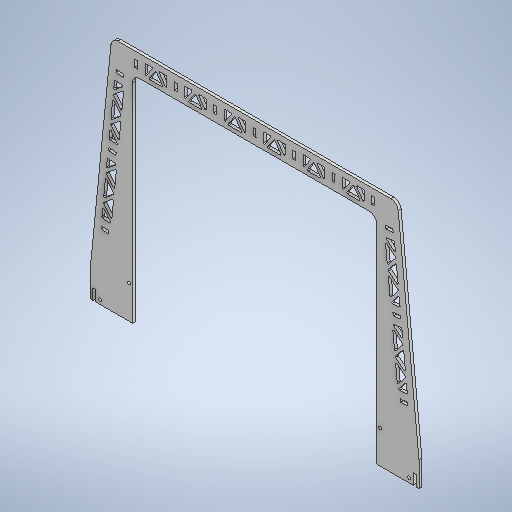
# Autodesk Inventor part: GateBrigeSide
Saved by Autodesk Inventor 2025.1 (Build 291241000, 241)
## iProperties
Created: 2025-03-30
Part Number: GateBrigeSide
Material: Všeobecné
Document SubType Name: Modeling
Designer: 42060
Density: 1 g/cm^3
Appearance: Výchozí
Author: 42060
Autodesk Inventor part; units mm, degrees
ref_plane "YZ Plane" through (0, 0, 0) normal (1, 0, 0) x (0, 1, 0)
ref_plane "XZ Plane" through (0, 0, 0) normal (0, 1, 0) x (-1, 0, 0)
ref_plane "XY Plane" through (0, 0, 0) normal (0, 0, 1) x (1, 0, 0)
sketch "Náčrt1" plane through (0, 0, 0) normal (0, 0, 1) x (1, 0, 0)
  line L0 (0, 0) -> (-160, 0)
  line L1 (-170, -10) -> (-170, -300)
  line L2 (-229, -300) -> (-229, -265.3)
  line L3 (-190.0509, 30) -> (0, 30)
  line L4 (0, 30) -> (0, 0)
  line L5 (-203.7, -249) -> (-170, -249)
  line L6 (-170, -249) -> (-170, -299)
  line L7 (-170, -299) -> (-220, -299)
  line L8 (-220, -299) -> (-220, -265.3)
  line L9 (-220, -265.3) -> (-203.7, -249)
  line L10 (-220, -299) -> (-170, -249) construction
  circle A0 centre (-215, -294) radius 2.1
  circle A1 centre (-175, -254) radius 2.1
  arc A2 (-160, 0) -> (-170, -10) centre (-160, -10) ccw
  line L11 (-200, 21.0077) -> (-229, -265.3)
  arc A3 (-190.0509, 30) -> (-200, 21.0077) centre (-190.0509, 20) ccw
  line L12 (-225, -300) -> (-225, -285)
  line L13 (-225, -285) -> (-221, -285)
  line L14 (-221, -285) -> (-221, -300)
  line L15 (-170, -300) -> (-221, -300)
  line L16 (-225, -300) -> (-229, -300)
  line L17 (-2, 10) -> (2, 10)
  line L18 (2, 10) -> (2, 20)
  line L19 (2, 20) -> (-2, 20)
  line L20 (-2, 20) -> (-2, 10)
  line L21 (-57, 20) -> (-57, 10)
  line L22 (-53, 20) -> (-57, 20)
  line L23 (-53, 10) -> (-53, 20)
  line L24 (-57, 10) -> (-53, 10)
  line L25 (-112, 20) -> (-112, 10)
  line L26 (-108, 20) -> (-112, 20)
  line L27 (-108, 10) -> (-108, 20)
  line L28 (-112, 10) -> (-108, 10)
  line L29 (-167, 20) -> (-167, 10)
  line L30 (-163, 20) -> (-167, 20)
  line L31 (-163, 10) -> (-163, 20)
  line L32 (-167, 10) -> (-163, 10)
  line L33 (-192.5844, -5.0126) -> (-182.6353, -6.0204)
  line L34 (-182.6353, -6.0204) -> (-183.0384, -10)
  line L35 (-183.0384, -10) -> (-192.9875, -8.9923)
  line L36 (-192.9875, -8.9923) -> (-192.5844, -5.0126)
  line L37 (-193.1158, -109.4909) -> (-203.0649, -108.4832)
  line L38 (-192.7127, -105.5113) -> (-193.1158, -109.4909)
  line L39 (-203.0649, -108.4832) -> (-202.6618, -104.5036)
  line L40 (-202.6618, -104.5036) -> (-192.7127, -105.5113)
  line L41 (-203.1932, -208.9819) -> (-213.1423, -207.9741)
  line L42 (-202.7901, -205.0022) -> (-203.1932, -208.9819)
  line L43 (-213.1423, -207.9741) -> (-212.7392, -203.9945)
  line L44 (-212.7392, -203.9945) -> (-202.7901, -205.0022)
  line L45 (0, 0) -> (160, 0)
  line L46 (170, -10) -> (170, -300)
  line L47 (229, -300) -> (229, -265.3)
  line L48 (190.0509, 30) -> (0, 30)
  line L49 (203.7, -249) -> (170, -249)
  line L50 (170, -249) -> (170, -299)
  line L51 (170, -299) -> (220, -299)
  line L52 (220, -299) -> (220, -265.3)
  line L53 (220, -265.3) -> (203.7, -249)
  line L54 (220, -299) -> (170, -249) construction
  circle A4 centre (215, -294) radius 2.1
  circle A5 centre (175, -254) radius 2.1
  arc A6 (170, -10) -> (160, 0) centre (160, -10) ccw
  line L55 (200, 21.0077) -> (229, -265.3)
  arc A7 (200, 21.0077) -> (190.0509, 30) centre (190.0509, 20) ccw
  line L56 (225, -300) -> (225, -285)
  line L57 (225, -285) -> (221, -285)
  line L58 (221, -285) -> (221, -300)
  line L59 (170, -300) -> (221, -300)
  line L60 (225, -300) -> (229, -300)
  line L61 (2, 10) -> (-2, 10)
  line L62 (-2, 10) -> (-2, 20)
  line L63 (-2, 20) -> (2, 20)
  line L64 (2, 20) -> (2, 10)
  line L65 (57, 20) -> (57, 10)
  line L66 (53, 20) -> (57, 20)
  line L67 (53, 10) -> (53, 20)
  line L68 (57, 10) -> (53, 10)
  line L69 (112, 20) -> (112, 10)
  line L70 (108, 20) -> (112, 20)
  line L71 (108, 10) -> (108, 20)
  line L72 (112, 10) -> (108, 10)
  line L73 (167, 20) -> (167, 10)
  line L74 (163, 20) -> (167, 20)
  line L75 (163, 10) -> (163, 20)
  line L76 (167, 10) -> (163, 10)
  line L77 (192.5844, -5.0126) -> (182.6353, -6.0204)
  line L78 (182.6353, -6.0204) -> (183.0384, -10)
  line L79 (183.0384, -10) -> (192.9875, -8.9923)
  line L80 (192.9875, -8.9923) -> (192.5844, -5.0126)
  line L81 (193.1158, -109.4909) -> (203.0649, -108.4832)
  line L82 (192.7127, -105.5113) -> (193.1158, -109.4909)
  line L83 (203.0649, -108.4832) -> (202.6618, -104.5036)
  line L84 (202.6618, -104.5036) -> (192.7127, -105.5113)
  line L85 (203.1932, -208.9819) -> (213.1423, -207.9741)
  line L86 (202.7901, -205.0022) -> (203.1932, -208.9819)
  line L87 (213.1423, -207.9741) -> (212.7392, -203.9945)
  line L88 (212.7392, -203.9945) -> (202.7901, -205.0022)
  line L89 (-36.6095, 7.1947) -> (-28.3278, 19.4124)
  line L90 (-26.6722, 19.4124) -> (-18.3905, 7.1947)
  line L91 (-19.2183, 5.6336) -> (-35.7817, 5.6336)
  line L92 (-22.6095, 20.5478) -> (-14.3278, 8.33)
  line L93 (-12.5, 8.8911) -> (-12.5, 21.1089)
  line L94 (-13.5, 22.1089) -> (-21.7817, 22.1089)
  line L95 (-32.3905, 20.5478) -> (-40.6722, 8.33)
  line L96 (-42.5, 8.8911) -> (-42.5, 21.1089)
  line L97 (-41.5, 22.1089) -> (-33.2183, 22.1089)
  line L98 (-53, 15) -> (-2, 15) construction
  arc A8 (-41.5, 22.1089) -> (-42.5, 21.1089) centre (-41.5, 21.1089) ccw
  arc A9 (-32.3905, 20.5478) -> (-33.2183, 22.1089) centre (-33.2183, 21.1089) ccw
  arc A10 (-42.5, 8.8911) -> (-40.6722, 8.33) centre (-41.5, 8.8911) ccw
  arc A11 (-36.6095, 7.1947) -> (-35.7817, 5.6336) centre (-35.7817, 6.6336) ccw
  arc A12 (-19.2183, 5.6336) -> (-18.3905, 7.1947) centre (-19.2183, 6.6336) ccw
  arc A13 (-26.6722, 19.4124) -> (-28.3278, 19.4124) centre (-27.5, 18.8514) ccw
  arc A14 (-21.7817, 22.1089) -> (-22.6095, 20.5478) centre (-21.7817, 21.1089) ccw
  arc A15 (-12.5, 21.1089) -> (-13.5, 22.1089) centre (-13.5, 21.1089) ccw
  arc A16 (-14.3278, 8.33) -> (-12.5, 8.8911) centre (-13.5, 8.8911) ccw
  arc A17 (-81.6722, 19.4124) -> (-83.3278, 19.4124) centre (-82.5, 18.8514) ccw
  line L99 (-91.6095, 7.1947) -> (-83.3278, 19.4124)
  line L100 (-68.5, 22.1089) -> (-76.7817, 22.1089)
  arc A18 (-67.5, 21.1089) -> (-68.5, 22.1089) centre (-68.5, 21.1089) ccw
  line L101 (-81.6722, 19.4124) -> (-73.3905, 7.1947)
  arc A19 (-74.2183, 5.6336) -> (-73.3905, 7.1947) centre (-74.2183, 6.6336) ccw
  line L102 (-77.6095, 20.5478) -> (-69.3278, 8.33)
  line L103 (-74.2183, 5.6336) -> (-90.7817, 5.6336)
  arc A20 (-69.3278, 8.33) -> (-67.5, 8.8911) centre (-68.5, 8.8911) ccw
  line L104 (-108, 15) -> (-57, 15) construction
  arc A21 (-96.5, 22.1089) -> (-97.5, 21.1089) centre (-96.5, 21.1089) ccw
  arc A22 (-97.5, 8.8911) -> (-95.6722, 8.33) centre (-96.5, 8.8911) ccw
  arc A23 (-91.6095, 7.1947) -> (-90.7817, 5.6336) centre (-90.7817, 6.6336) ccw
  arc A24 (-87.3905, 20.5478) -> (-88.2183, 22.1089) centre (-88.2183, 21.1089) ccw
  line L105 (-67.5, 8.8911) -> (-67.5, 21.1089)
  arc A25 (-76.7817, 22.1089) -> (-77.6095, 20.5478) centre (-76.7817, 21.1089) ccw
  line L106 (-96.5, 22.1089) -> (-88.2183, 22.1089)
  line L107 (-87.3905, 20.5478) -> (-95.6722, 8.33)
  line L108 (-97.5, 8.8911) -> (-97.5, 21.1089)
  arc A26 (-136.6722, 19.4124) -> (-138.3278, 19.4124) centre (-137.5, 18.8514) ccw
  line L109 (-146.6095, 7.1947) -> (-138.3278, 19.4124)
  line L110 (-123.5, 22.1089) -> (-131.7817, 22.1089)
  arc A27 (-122.5, 21.1089) -> (-123.5, 22.1089) centre (-123.5, 21.1089) ccw
  line L111 (-136.6722, 19.4124) -> (-128.3905, 7.1947)
  arc A28 (-129.2183, 5.6336) -> (-128.3905, 7.1947) centre (-129.2183, 6.6336) ccw
  line L112 (-132.6095, 20.5478) -> (-124.3278, 8.33)
  line L113 (-129.2183, 5.6336) -> (-145.7817, 5.6336)
  arc A29 (-124.3278, 8.33) -> (-122.5, 8.8911) centre (-123.5, 8.8911) ccw
  line L114 (-163, 15) -> (-112, 15) construction
  arc A30 (-151.5, 22.1089) -> (-152.5, 21.1089) centre (-151.5, 21.1089) ccw
  arc A31 (-152.5, 8.8911) -> (-150.6722, 8.33) centre (-151.5, 8.8911) ccw
  arc A32 (-146.6095, 7.1947) -> (-145.7817, 5.6336) centre (-145.7817, 6.6336) ccw
  arc A33 (-142.3905, 20.5478) -> (-143.2183, 22.1089) centre (-143.2183, 21.1089) ccw
  line L115 (-122.5, 8.8911) -> (-122.5, 21.1089)
  arc A34 (-131.7817, 22.1089) -> (-132.6095, 20.5478) centre (-131.7817, 21.1089) ccw
  line L116 (-151.5, 22.1089) -> (-143.2183, 22.1089)
  line L117 (-142.3905, 20.5478) -> (-150.6722, 8.33)
  line L118 (-152.5, 8.8911) -> (-152.5, 21.1089)
  line L119 (-193.9599, -18.9449) -> (-184.0815, -19.9455)
  line L120 (-183.55, -21.7152) -> (-194.429, -30.593)
  line L121 (-196.0562, -29.7175) -> (-195.0556, -19.8391)
  line L122 (-182.493, -28.2188) -> (-184.6957, -49.9654)
  line L123 (-186.4653, -50.4969) -> (-196.2373, -38.5222)
  line L124 (-196.0948, -37.1152) -> (-184.1201, -27.3432)
  line L125 (-195.9132, -45.2459) -> (-186.1413, -57.2206)
  line L126 (-186.2838, -58.6276) -> (-198.2584, -68.3996)
  line L127 (-199.8856, -67.524) -> (-197.6829, -45.7774)
  line L128 (-187.9495, -65.1498) -> (-199.9242, -74.9217)
  line L129 (-200.0667, -76.3288) -> (-190.2947, -88.3034)
  line L130 (-188.5251, -87.7719) -> (-186.3224, -66.0253)
  line L131 (-199.7426, -83.0525) -> (-190.8648, -93.9315)
  line L132 (-191.7403, -95.5586) -> (-201.6187, -94.558)
  line L133 (-202.5129, -93.4624) -> (-201.5123, -83.584)
  line L134 (-189.0207, -19.4452) -> (-188.013, -9.4961)
  arc A35 (-193.9599, -18.9449) -> (-195.0556, -19.8391) centre (-194.0607, -19.9398) ccw
  arc A36 (-183.55, -21.7152) -> (-184.0815, -19.9455) centre (-184.1823, -20.9404) ccw
  arc A37 (-196.0562, -29.7175) -> (-194.429, -30.593) centre (-195.0613, -29.8182) ccw
  arc A38 (-196.0948, -37.1152) -> (-196.2373, -38.5222) centre (-195.4625, -37.89) ccw
  arc A39 (-186.4653, -50.4969) -> (-184.6957, -49.9654) centre (-185.6906, -49.8646) ccw
  arc A40 (-182.493, -28.2188) -> (-184.1201, -27.3432) centre (-183.4879, -28.118) ccw
  arc A41 (-195.9132, -45.2459) -> (-197.6829, -45.7774) centre (-196.688, -45.8782) ccw
  arc A42 (-186.2838, -58.6276) -> (-186.1413, -57.2206) centre (-186.916, -57.8528) ccw
  arc A43 (-199.8856, -67.524) -> (-198.2584, -68.3996) centre (-198.8907, -67.6248) ccw
  arc A44 (-199.9242, -74.9217) -> (-200.0667, -76.3288) centre (-199.2919, -75.6965) ccw
  arc A45 (-190.2947, -88.3034) -> (-188.5251, -87.7719) centre (-189.52, -87.6712) ccw
  arc A46 (-186.3224, -66.0253) -> (-187.9495, -65.1498) centre (-187.3173, -65.9246) ccw
  arc A47 (-199.7426, -83.0525) -> (-201.5123, -83.584) centre (-200.5174, -83.6847) ccw
  arc A48 (-202.5129, -93.4624) -> (-201.6187, -94.558) centre (-201.518, -93.5631) ccw
  arc A49 (-191.7403, -95.5586) -> (-190.8648, -93.9315) centre (-191.6396, -94.5637) ccw
  arc A50 (-212.5903, -192.9533) -> (-211.6961, -194.049) centre (-211.5954, -193.0541) ccw
  line L135 (-201.8177, -195.0496) -> (-211.6961, -194.049)
  arc A51 (-201.8177, -195.0496) -> (-200.9422, -193.4224) centre (-201.717, -194.0546) ccw
  arc A52 (-200.3721, -187.7943) -> (-198.6025, -187.2629) centre (-199.5974, -187.1621) ccw
  line L136 (-209.82, -182.5434) -> (-200.9422, -193.4224)
  line L137 (-212.5903, -192.9533) -> (-211.5897, -183.0749)
  arc A53 (-209.82, -182.5434) -> (-211.5897, -183.0749) centre (-210.5948, -183.1757) ccw
  line L138 (-198.0269, -164.6407) -> (-210.0016, -174.4127)
  line L139 (-210.1441, -175.8197) -> (-200.3721, -187.7943)
  line L140 (-198.6025, -187.2629) -> (-196.3998, -165.5163)
  arc A54 (-210.0016, -174.4127) -> (-210.1441, -175.8197) centre (-209.3693, -175.1874) ccw
  arc A55 (-209.963, -167.0149) -> (-208.3358, -167.8905) centre (-208.9681, -167.1157) ccw
  arc A56 (-196.3998, -165.5163) -> (-198.0269, -164.6407) centre (-197.3947, -165.4155) ccw
  line L141 (-205.9906, -144.7369) -> (-196.2187, -156.7115)
  arc A57 (-196.3612, -158.1185) -> (-196.2187, -156.7115) centre (-196.9934, -157.3438) ccw
  line L142 (-209.963, -167.0149) -> (-207.7603, -145.2684)
  line L143 (-196.3612, -158.1185) -> (-208.3358, -167.8905)
  arc A58 (-196.5427, -149.9878) -> (-194.7731, -149.4563) centre (-195.768, -149.3555) ccw
  arc A59 (-205.9906, -144.7369) -> (-207.7603, -145.2684) centre (-206.7654, -145.3691) ccw
  line L144 (-196.5427, -149.9878) -> (-206.3147, -138.0131)
  arc A60 (-206.1722, -136.6061) -> (-206.3147, -138.0131) centre (-205.5399, -137.3809) ccw
  arc A61 (-206.1336, -129.2084) -> (-204.5064, -130.0839) centre (-205.1387, -129.3092) ccw
  line L145 (-192.5703, -127.7097) -> (-194.7731, -149.4563)
  line L146 (-206.1722, -136.6061) -> (-194.1975, -126.8342)
  arc A62 (-192.5703, -127.7097) -> (-194.1975, -126.8342) centre (-193.5653, -127.6089) ccw
  arc A63 (-193.6274, -121.2061) -> (-194.1589, -119.4364) centre (-194.2597, -120.4314) ccw
  line L147 (-199.0981, -118.9362) -> (-198.0904, -108.9871)
  line L148 (-204.0373, -118.4359) -> (-194.1589, -119.4364)
  arc A64 (-204.0373, -118.4359) -> (-205.133, -119.33) centre (-204.1381, -119.4308) ccw
  line L149 (-193.6274, -121.2061) -> (-204.5064, -130.0839)
  line L150 (-206.1336, -129.2084) -> (-205.133, -119.33)
  line L151 (36.6095, 7.1947) -> (28.3278, 19.4124)
  line L152 (26.6722, 19.4124) -> (18.3905, 7.1947)
  line L153 (19.2183, 5.6336) -> (35.7817, 5.6336)
  line L154 (22.6095, 20.5478) -> (14.3278, 8.33)
  line L155 (12.5, 8.8911) -> (12.5, 21.1089)
  line L156 (13.5, 22.1089) -> (21.7817, 22.1089)
  line L157 (32.3905, 20.5478) -> (40.6722, 8.33)
  line L158 (42.5, 8.8911) -> (42.5, 21.1089)
  line L159 (41.5, 22.1089) -> (33.2183, 22.1089)
  line L160 (53, 15) -> (2, 15) construction
  arc A65 (42.5, 21.1089) -> (41.5, 22.1089) centre (41.5, 21.1089) ccw
  arc A66 (33.2183, 22.1089) -> (32.3905, 20.5478) centre (33.2183, 21.1089) ccw
  arc A67 (40.6722, 8.33) -> (42.5, 8.8911) centre (41.5, 8.8911) ccw
  arc A68 (35.7817, 5.6336) -> (36.6095, 7.1947) centre (35.7817, 6.6336) ccw
  arc A69 (18.3905, 7.1947) -> (19.2183, 5.6336) centre (19.2183, 6.6336) ccw
  arc A70 (28.3278, 19.4124) -> (26.6722, 19.4124) centre (27.5, 18.8514) ccw
  arc A71 (22.6095, 20.5478) -> (21.7817, 22.1089) centre (21.7817, 21.1089) ccw
  arc A72 (13.5, 22.1089) -> (12.5, 21.1089) centre (13.5, 21.1089) ccw
  arc A73 (12.5, 8.8911) -> (14.3278, 8.33) centre (13.5, 8.8911) ccw
  line L161 (67.5, 8.8911) -> (67.5, 21.1089)
  line L162 (96.5, 22.1089) -> (88.2183, 22.1089)
  arc A74 (97.5, 21.1089) -> (96.5, 22.1089) centre (96.5, 21.1089) ccw
  line L163 (97.5, 8.8911) -> (97.5, 21.1089)
  arc A75 (95.6722, 8.33) -> (97.5, 8.8911) centre (96.5, 8.8911) ccw
  arc A76 (67.5, 8.8911) -> (69.3278, 8.33) centre (68.5, 8.8911) ccw
  arc A77 (68.5, 22.1089) -> (67.5, 21.1089) centre (68.5, 21.1089) ccw
  arc A78 (88.2183, 22.1089) -> (87.3905, 20.5478) centre (88.2183, 21.1089) ccw
  arc A79 (83.3278, 19.4124) -> (81.6722, 19.4124) centre (82.5, 18.8514) ccw
  line L164 (87.3905, 20.5478) -> (95.6722, 8.33)
  line L165 (91.6095, 7.1947) -> (83.3278, 19.4124)
  arc A80 (77.6095, 20.5478) -> (76.7817, 22.1089) centre (76.7817, 21.1089) ccw
  arc A81 (90.7817, 5.6336) -> (91.6095, 7.1947) centre (90.7817, 6.6336) ccw
  line L166 (108, 15) -> (57, 15) construction
  line L167 (68.5, 22.1089) -> (76.7817, 22.1089)
  line L168 (77.6095, 20.5478) -> (69.3278, 8.33)
  line L169 (81.6722, 19.4124) -> (73.3905, 7.1947)
  arc A82 (73.3905, 7.1947) -> (74.2183, 5.6336) centre (74.2183, 6.6336) ccw
  line L170 (74.2183, 5.6336) -> (90.7817, 5.6336)
  line L171 (122.5, 8.8911) -> (122.5, 21.1089)
  line L172 (151.5, 22.1089) -> (143.2183, 22.1089)
  arc A83 (152.5, 21.1089) -> (151.5, 22.1089) centre (151.5, 21.1089) ccw
  line L173 (152.5, 8.8911) -> (152.5, 21.1089)
  arc A84 (150.6722, 8.33) -> (152.5, 8.8911) centre (151.5, 8.8911) ccw
  arc A85 (122.5, 8.8911) -> (124.3278, 8.33) centre (123.5, 8.8911) ccw
  arc A86 (123.5, 22.1089) -> (122.5, 21.1089) centre (123.5, 21.1089) ccw
  arc A87 (143.2183, 22.1089) -> (142.3905, 20.5478) centre (143.2183, 21.1089) ccw
  arc A88 (138.3278, 19.4124) -> (136.6722, 19.4124) centre (137.5, 18.8514) ccw
  line L174 (142.3905, 20.5478) -> (150.6722, 8.33)
  line L175 (146.6095, 7.1947) -> (138.3278, 19.4124)
  arc A89 (132.6095, 20.5478) -> (131.7817, 22.1089) centre (131.7817, 21.1089) ccw
  arc A90 (145.7817, 5.6336) -> (146.6095, 7.1947) centre (145.7817, 6.6336) ccw
  line L176 (163, 15) -> (112, 15) construction
  line L177 (123.5, 22.1089) -> (131.7817, 22.1089)
  line L178 (132.6095, 20.5478) -> (124.3278, 8.33)
  line L179 (136.6722, 19.4124) -> (128.3905, 7.1947)
  arc A91 (128.3905, 7.1947) -> (129.2183, 5.6336) centre (129.2183, 6.6336) ccw
  line L180 (129.2183, 5.6336) -> (145.7817, 5.6336)
  line L181 (193.9599, -18.9449) -> (184.0815, -19.9455)
  line L182 (183.55, -21.7152) -> (194.429, -30.593)
  line L183 (196.0562, -29.7175) -> (195.0556, -19.8391)
  line L184 (182.493, -28.2188) -> (184.6957, -49.9654)
  line L185 (186.4653, -50.4969) -> (196.2373, -38.5222)
  line L186 (196.0948, -37.1152) -> (184.1201, -27.3432)
  line L187 (195.9132, -45.2459) -> (186.1413, -57.2206)
  line L188 (186.2838, -58.6276) -> (198.2584, -68.3996)
  line L189 (199.8856, -67.524) -> (197.6829, -45.7774)
  line L190 (187.9495, -65.1498) -> (199.9242, -74.9217)
  line L191 (200.0667, -76.3288) -> (190.2947, -88.3034)
  line L192 (188.5251, -87.7719) -> (186.3224, -66.0253)
  line L193 (199.7426, -83.0525) -> (190.8648, -93.9315)
  line L194 (191.7403, -95.5586) -> (201.6187, -94.558)
  line L195 (202.5129, -93.4624) -> (201.5123, -83.584)
  line L196 (189.0207, -19.4452) -> (188.013, -9.4961)
  arc A92 (195.0556, -19.8391) -> (193.9599, -18.9449) centre (194.0607, -19.9398) ccw
  arc A93 (184.0815, -19.9455) -> (183.55, -21.7152) centre (184.1823, -20.9404) ccw
  arc A94 (194.429, -30.593) -> (196.0562, -29.7175) centre (195.0613, -29.8182) ccw
  arc A95 (196.2373, -38.5222) -> (196.0948, -37.1152) centre (195.4625, -37.89) ccw
  arc A96 (184.6957, -49.9654) -> (186.4653, -50.4969) centre (185.6906, -49.8646) ccw
  arc A97 (184.1201, -27.3432) -> (182.493, -28.2188) centre (183.4879, -28.118) ccw
  arc A98 (197.6829, -45.7774) -> (195.9132, -45.2459) centre (196.688, -45.8782) ccw
  arc A99 (186.1413, -57.2206) -> (186.2838, -58.6276) centre (186.916, -57.8528) ccw
  arc A100 (198.2584, -68.3996) -> (199.8856, -67.524) centre (198.8907, -67.6248) ccw
  arc A101 (200.0667, -76.3288) -> (199.9242, -74.9217) centre (199.2919, -75.6965) ccw
  arc A102 (188.5251, -87.7719) -> (190.2947, -88.3034) centre (189.52, -87.6712) ccw
  arc A103 (187.9495, -65.1498) -> (186.3224, -66.0253) centre (187.3173, -65.9246) ccw
  arc A104 (201.5123, -83.584) -> (199.7426, -83.0525) centre (200.5174, -83.6847) ccw
  arc A105 (201.6187, -94.558) -> (202.5129, -93.4624) centre (201.518, -93.5631) ccw
  arc A106 (190.8648, -93.9315) -> (191.7403, -95.5586) centre (191.6396, -94.5637) ccw
  arc A107 (194.1589, -119.4364) -> (193.6274, -121.2061) centre (194.2597, -120.4314) ccw
  arc A108 (194.1975, -126.8342) -> (192.5703, -127.7097) centre (193.5653, -127.6089) ccw
  line L197 (204.0373, -118.4359) -> (194.1589, -119.4364)
  line L198 (193.6274, -121.2061) -> (204.5064, -130.0839)
  line L199 (206.1336, -129.2084) -> (205.133, -119.33)
  line L200 (206.1722, -136.6061) -> (194.1975, -126.8342)
  arc A109 (205.133, -119.33) -> (204.0373, -118.4359) centre (204.1381, -119.4308) ccw
  arc A110 (204.5064, -130.0839) -> (206.1336, -129.2084) centre (205.1387, -129.3092) ccw
  line L201 (192.5703, -127.7097) -> (194.7731, -149.4563)
  arc A111 (207.7603, -145.2684) -> (205.9906, -144.7369) centre (206.7654, -145.3691) ccw
  line L202 (196.5427, -149.9878) -> (206.3147, -138.0131)
  arc A112 (206.3147, -138.0131) -> (206.1722, -136.6061) centre (205.5399, -137.3809) ccw
  arc A113 (194.7731, -149.4563) -> (196.5427, -149.9878) centre (195.768, -149.3555) ccw
  line L203 (205.9906, -144.7369) -> (196.2187, -156.7115)
  arc A114 (196.2187, -156.7115) -> (196.3612, -158.1185) centre (196.9934, -157.3438) ccw
  arc A115 (198.0269, -164.6407) -> (196.3998, -165.5163) centre (197.3947, -165.4155) ccw
  line L204 (196.3612, -158.1185) -> (208.3358, -167.8905)
  arc A116 (208.3358, -167.8905) -> (209.963, -167.0149) centre (208.9681, -167.1157) ccw
  line L205 (209.963, -167.0149) -> (207.7603, -145.2684)
  arc A117 (200.9422, -193.4224) -> (201.8177, -195.0496) centre (201.717, -194.0546) ccw
  arc A118 (211.6961, -194.049) -> (212.5903, -192.9533) centre (211.5954, -193.0541) ccw
  arc A119 (198.6025, -187.2629) -> (200.3721, -187.7943) centre (199.5974, -187.1621) ccw
  line L206 (212.5903, -192.9533) -> (211.5897, -183.0749)
  line L207 (209.82, -182.5434) -> (200.9422, -193.4224)
  arc A120 (211.5897, -183.0749) -> (209.82, -182.5434) centre (210.5948, -183.1757) ccw
  line L208 (210.1441, -175.8197) -> (200.3721, -187.7943)
  arc A121 (210.1441, -175.8197) -> (210.0016, -174.4127) centre (209.3693, -175.1874) ccw
  line L209 (198.6025, -187.2629) -> (196.3998, -165.5163)
  line L210 (198.0269, -164.6407) -> (210.0016, -174.4127)
  line L211 (201.8177, -195.0496) -> (211.6961, -194.049)
  point P0 (2, 15)
  point P1 (0, 15)
  point P2 (0, 10)
  point P3 (-55, 10)
  point P4 (-110, 10)
  point P5 (-165, 10)
  point P6 (55, 10)
  point P7 (108, 15)
  point P8 (110, 10)
  point P9 (163, 15)
  point P10 (165, 10)
  point P11 (-27.5, 20.6336)
  point P12 (-12.5, 5.6336)
  point P13 (-31.3323, 22.1089)
  point P14 (-42.5, 22.1089)
  point P15 (-27.5, 5.6336)
  point P16 (-27.5, 15)
  point P17 (-12.5, 15)
  point P18 (-2, 15)
  point P19 (-82.5, 20.6336)
  point P20 (-82.5, 15)
  point P21 (-82.5, 5.6336)
  point P22 (-86.3323, 22.1089)
  point P23 (-97.5, 22.1089)
  point P24 (-67.5, 5.6336)
  point P25 (-67.5, 15)
  point P26 (-137.5, 20.6336)
  point P27 (-137.5, 15)
  point P28 (-137.5, 5.6336)
  point P29 (-141.3323, 22.1089)
  point P30 (-152.5, 22.1089)
  point P31 (-122.5, 5.6336)
  point P32 (-122.5, 15)
  point P33 (-194.9548, -18.8442)
  point P34 (-181.6796, -20.1888)
  point P35 (-196.2995, -32.1194)
  point P36 (-182.2497, -25.8169)
  point P37 (-184.9389, -52.3673)
  point P38 (-196.8695, -37.7474)
  point P39 (-197.4396, -43.3755)
  point P40 (-185.509, -57.9954)
  point P41 (-200.1289, -69.9259)
  point P42 (-186.0791, -63.6234)
  point P43 (-200.6989, -75.554)
  point P44 (-188.7684, -90.1739)
  point P45 (-201.269, -81.1821)
  point P46 (-189.3384, -95.8019)
  point P47 (-202.6136, -94.4573)
  point P48 (-212.691, -193.9482)
  point P49 (-199.4158, -195.2928)
  point P50 (-198.8458, -189.6648)
  point P51 (-211.3464, -180.673)
  point P52 (-210.7763, -175.0449)
  point P53 (-210.2063, -169.4169)
  point P54 (-196.1565, -163.1143)
  point P55 (-195.5864, -157.4863)
  point P56 (-195.0163, -151.8582)
  point P57 (-207.517, -142.8664)
  point P58 (-206.9469, -137.2384)
  point P59 (-206.3769, -131.6103)
  point P60 (-192.3271, -125.3078)
  point P61 (-191.757, -119.6797)
  point P62 (-205.0322, -118.3351)
  point P63 (27.5, 20.6336)
  point P64 (12.5, 5.6336)
  point P65 (31.3323, 22.1089)
  point P66 (42.5, 22.1089)
  point P67 (27.5, 5.6336)
  point P68 (27.5, 15)
  point P69 (12.5, 15)
  point P70 (67.5, 5.6336)
  point P71 (67.5, 15)
  point P72 (82.5, 20.6336)
  point P73 (86.3323, 22.1089)
  point P74 (97.5, 22.1089)
  point P75 (82.5, 15)
  point P76 (82.5, 5.6336)
  point P77 (122.5, 5.6336)
  point P78 (122.5, 15)
  point P79 (137.5, 20.6336)
  point P80 (141.3323, 22.1089)
  point P81 (152.5, 22.1089)
  point P82 (137.5, 15)
  point P83 (137.5, 5.6336)
  point P84 (194.9548, -18.8442)
  point P85 (181.6796, -20.1888)
  point P86 (196.2995, -32.1194)
  point P87 (182.2497, -25.8169)
  point P88 (184.9389, -52.3673)
  point P89 (196.8695, -37.7474)
  point P90 (197.4396, -43.3755)
  point P91 (185.509, -57.9954)
  point P92 (200.1289, -69.9259)
  point P93 (186.0791, -63.6234)
  point P94 (200.6989, -75.554)
  point P95 (188.7684, -90.1739)
  point P96 (201.269, -81.1821)
  point P97 (189.3384, -95.8019)
  point P98 (202.6136, -94.4573)
  point P99 (191.757, -119.6797)
  point P100 (192.3271, -125.3078)
  point P101 (199.0981, -118.9362)
  point P102 (205.0322, -118.3351)
  point P103 (206.3769, -131.6103)
  point P104 (206.9469, -137.2384)
  point P105 (195.0163, -151.8582)
  point P106 (207.517, -142.8664)
  point P107 (195.5864, -157.4863)
  point P108 (196.1565, -163.1143)
  point P109 (210.2063, -169.4169)
  point P110 (212.691, -193.9482)
  point P111 (199.4158, -195.2928)
  point P112 (198.8458, -189.6648)
  point P113 (210.7763, -175.0449)
  point P114 (211.3464, -180.673)
  dimension "d0" = 50
  dimension "d1" = 50
  dimension "d3" = 33.7
  dimension "d4" = 45
  dimension "d5" = 0
  dimension "d6" = 4.2
  dimension "d7" = 5
  dimension "d8" = 5
  dimension "d10" = 170
  dimension "d12" = 30
  dimension "d14" = 10
  dimension "d16" = 15
  dimension "d17" = 1
  dimension "d18" = 4
  dimension "d19" = 1
  dimension "d20" = 4
  dimension "d21" = 300
  dimension "d22" = 30
  dimension "d25" = 4
  dimension "d26" = 10
  dimension "d29" = 55
  dimension "d34" = 4
  dimension "d35" = 10
  dimension "d36" = 10
  dimension "d39" = 100
  dimension "d46" = 4
  dimension "d47" = 4
  dimension "d50" = 15
  dimension "d51" = 30
  dimension "d52" = 1
  dimension "d55" = 55
  dimension "d60" = 10
  dimension "d61" = 10
  dimension "d63" = 4
  dimension "d64" = 4
  dimension "d65" = 4
  dimension "d66" = 4
  dimension "d67" = 1
  dimension "d70" = 100
  dimension "d77" = 55
  dimension "d84" = 100
  constraints: 424 end point, 236 point on circle, 210 point on line, 152 symmetric about line, 122 centre point, 52 tangent, 24 equal radius, 18 perpendicular, 17 parallel, 9 midpoint, 8 horizontal, 7 collinear, 5 horizontal alignment, 4 equal length, 3 vertical alignment, 1 vertical, 481 other
  measures "d0" distance of L5.end L6.end
  measures "d1" distance of L6.end L7.end
  measures "d3" distance of L5.start L5.end
  measures "d4" angle of L5 L9
  measures "d5" distance between parallel lines of L1 L6
  measures "d6" diameter of A1
  measures "d7" distance from line of L5 A1.centre
  measures "d8" distance from line of L7 A0.centre
  measures "d10" distance between parallel lines of L1 L4
  measures "d12" distance between parallel lines of L0 L3
  measures "d14" radius of A3
  measures "d16" distance between parallel lines of L16 L13
  measures "d17" distance between parallel lines of L7 L15
  measures "d18" distance between parallel lines of L14 L12
  measures "d19" distance between parallel lines of L8 L14
  measures "d20" distance between parallel lines of L12 L2
  measures "d21" distance between parallel lines of L15 L0
  measures "d22" distance from line of L11.start L1
  measures "d25" distance of L18.end L19.end
  measures "d26" distance of L17.end L18.end
  measures "d29" distance of L19.end L21.start
  measures "d34" distance of L35.end L33.start
  measures "d35" distance of L33.start L33.end
  measures "d36" distance between parallel lines of L11 L36
  measures "d39" distance of L34.end L37.start
  measures "d46" distance between parallel lines of L89 L95
  measures "d47" distance between parallel lines of L92 L90
  measures "d50" distance from line of L91 point (-27.5, 20.634)
  measures "d51" distance between parallel lines of L93 L96
  measures "d52" radius of A8
  measures "d55" distance of point (-27.5, 20.634) point (-82.5, 20.634)
  measures "d60" distance between parallel lines of L35 L119
  measures "d61" distance between parallel lines of L132 L40
  measures "d63" distance between parallel lines of L124 L120
  measures "d64" distance between parallel lines of L125 L123
  measures "d65" distance between parallel lines of L128 L126
  measures "d66" distance between parallel lines of L129 L131
  measures "d67" radius of A35
  measures "d70" distance of point (-202.614, -94.457) point (-212.691, -193.948)
  measures "d77" distance of point (12.5, 5.634) point (67.5, 5.634)
  measures "d84" distance of point (181.68, -20.189) point (191.757, -119.68)
extrude "Vysunutí1" add sketch "Náčrt1" along normal blind 4 contours L0 A2 L1 L5 L9 L8 L7 L15 L14 L13 L12 L16 L2 L11 A3 L3 L4 L19 L20 L17 | L4 L17 L18 L19 L48 A7 L55 L47 L60 L56 L57 L58 L59 L46 L51 L52 L53 L49 A6 L45 | L1 L7 L8 L9 L5 | L49 L53 L52 L51 L46
equation "\"d25\" = d18"
equation "\"d34\" = d18"
equation "\"d35\" = d26"
equation "\"d36\" = d26"
equation "\"d44\" = d18"
